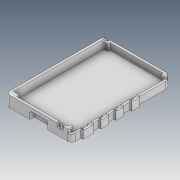
# Autodesk Inventor part: raspberry_pi_base
Saved by Autodesk Inventor 2020 (Build 240168000, 168)
## iProperties
Created: 2020-10-02
Part Number: raspberry_pi_base
Material: Generic
Document SubType Name: Modeling
Designer: DELL
Density: 1 g/cm^3
Appearance: Default
Mass: 14.8212 g
Surface Area: 156.939 cm^2
Volume: 14.8212 cm^3
Author: DELL
Autodesk Inventor part; units mm, degrees
ref_plane "YZ Plane" through (0, 0, 0) normal (1, 0, 0) x (0, 1, 0)
ref_plane "XZ Plane" through (0, 0, 0) normal (0, 1, 0) x (-1, 0, 0)
ref_plane "XY Plane" through (0, 0, 0) normal (0, 0, 1) x (1, 0, 0)
sketch "Sketch1" plane through (0, 0, 0) normal (0, 1, 0) x (-1, 0, 0)
  line L0 (-26.5, -44.85) -> (26.5, -44.85)
  line L1 (30, -41.35) -> (30, 41.35)
  line L2 (26.5, 44.85) -> (-26.5, 44.85)
  line L3 (-30, 41.35) -> (-30, -41.35)
  line L4 (-30, -44.85) -> (30, 44.85) construction
  line L5 (30, -44.85) -> (-30, 44.85) construction
  arc A0 (30, 41.35) -> (26.5, 44.85) centre (26.5, 41.35) ccw
  arc A1 (-26.5, 44.85) -> (-30, 41.35) centre (-26.5, 41.35) ccw
  arc A2 (26.5, -44.85) -> (30, -41.35) centre (26.5, -41.35) ccw
  arc A3 (-30, -41.35) -> (-26.5, -44.85) centre (-26.5, -41.35) ccw
  line L6 (-26.4, -46.85) -> (26.4, -46.85)
  line L7 (26.4, -46.85) -> (26.4, 0)
  line L8 (26.4, 0) -> (-26.4, 0)
  line L9 (-26.4, 0) -> (-26.4, -46.85)
  line L10 (-26.4, -46.85) -> (26.4, 0) construction
  line L11 (26.4, -46.85) -> (-26.4, 0) construction
  point P0 (0, 0)
  point P1 (0, -23.425)
  point P2 (0, 0)
  point P3 (0, 0)
  point P4 (0, -23.425)
  point P5 (0, 0)
  point P6 (-26.4, -44.85)
  point P7 (26.4, -44.85)
  dimension "d0" = 89.7
  dimension "d1" = 60
  dimension "d2" = 3.5
  dimension "d3" = 2
  dimension "d4" = 52.8
  constraints: 24 end point, 8 midpoint, 8 point on circle, 8 point on line, 8 tangent, 4 centre point, 4 parallel, 3 equal radius, 2 horizontal, 2 perpendicular, 1 coincident, 1 vertical alignment
  measures "d0" distance of L5.start L4.end
  measures "d1" distance of L4.start L5.start
  measures "d2" radius of A0
  measures "d3" distance between parallel lines of L0 L6
  measures "d4" distance of L6.start L6.end
extrude "Extrusion1" add sketch "Sketch1" along normal blind 2
sketch "Sketch2" plane through (30, 0, 41.35) normal (1, 0, 0) x (0, 0, -1)
  line L0 (0, 0) -> (82.7, 0) projected
  line L1 (14.7, 0) -> (5.1, 0)
  line L2 (5.1, 8.5) -> (5.1, 8)
  line L3 (5.1, 8) -> (14.7, 8)
  line L4 (14.7, 8) -> (14.7, 8.5)
  line L5 (28.4, 0) -> (21.4, 0)
  line L6 (21.4, 0) -> (21.4, 8)
  line L7 (21.4, 8) -> (28.4, 8)
  line L8 (28.4, 8) -> (28.4, 0)
  line L9 (42.1, 0) -> (35.1, 0)
  line L10 (35.1, 0) -> (35.1, 8)
  line L11 (35.1, 8) -> (42.1, 8)
  line L12 (42.1, 8) -> (42.1, 0)
  line L13 (56.4, 0) -> (49.7, 0)
  line L14 (49.7, 0) -> (49.7, 9)
  line L15 (49.7, 9) -> (56.4, 9)
  line L16 (56.4, 9) -> (56.4, 0)
  line L17 (-3.5, 0) -> (-3.5, 2) projected
  line L18 (5.1, 8) -> (14.7, 8)
  line L19 (14.7, 8) -> (14.7, 7)
  line L20 (13.2, 7) -> (6.6, 7)
  line L21 (5.1, 7) -> (5.1, 8)
  arc A0 (5.1, 8.5) -> (6.6, 7) centre (6.6, 8.5) ccw
  arc A1 (13.2, 7) -> (14.7, 8.5) centre (13.2, 8.5) ccw
  line L22 (5.1, 7) -> (5.1, 0)
  line L23 (14.7, 7) -> (14.7, 0)
  line L24 (21.4, 8) -> (28.4, 8)
  line L25 (28.4, 8) -> (28.4, 8.5)
  line L26 (26.9, 7) -> (22.9, 7)
  line L27 (21.4, 8.5) -> (21.4, 8)
  arc A2 (21.4, 8.5) -> (22.9, 7) centre (22.9, 8.5) ccw
  arc A3 (26.9, 7) -> (28.4, 8.5) centre (26.9, 8.5) ccw
  line L28 (35.1, 8) -> (42.1, 8)
  line L29 (42.1, 8) -> (42.1, 8.5)
  line L30 (40.6, 7) -> (36.6, 7)
  line L31 (35.1, 8.5) -> (35.1, 8)
  arc A4 (35.1, 8.5) -> (36.6, 7) centre (36.6, 8.5) ccw
  arc A5 (40.6, 7) -> (42.1, 8.5) centre (40.6, 8.5) ccw
  arc A6 (49.7, 9) -> (56.4, 9) centre (53.05, 11.1857) ccw
  point P0 (41.35, 0)
  point P1 (35.1858, 8)
  point P2 (35.1, 0)
  point P3 (42.0142, 8)
  point P4 (21.4858, 8)
  point P5 (28.3142, 8)
  point P6 (14.7, 8)
  point P7 (14.6142, 8)
  point P8 (5.1858, 8)
  point P9 (5.1, 0)
  dimension "d7" = 8
  dimension "d8" = 9.6
  dimension "d9" = 8.6
  dimension "d10" = 1
  dimension "d11" = 1.5
  dimension "d12" = 6.7
  dimension "d13" = 7
  dimension "d14" = 1.5
  dimension "d15" = 1
  dimension "d16" = 6.7
  dimension "d17" = 1.5
  dimension "d18" = 1
  dimension "d19" = 7.6
  dimension "d20" = 6.7
  dimension "d21" = 9
  dimension "d22" = 8
  constraints: 60 end point, 15 parallel, 14 point on circle, 12 point on line, 12 tangent, 7 centre point, 7 horizontal, 7 perpendicular, 6 collinear, 3 equal radius, 1 vertical
  measures "d7" distance between parallel lines of L0 L3
  measures "d8" distance of L2.end L3.end
  measures "d9" distance between parallel lines of L17 L2
  measures "d10" distance between parallel lines of L3 L20
  measures "d11" radius of A0
  measures "d12" distance between parallel lines of L6 L23
  measures "d13" distance of L6.end L7.end
  measures "d14" radius of A2
  measures "d15" distance between parallel lines of L24 L26
  measures "d16" distance between parallel lines of L8 L10
  measures "d17" radius of A4
  measures "d18" distance between parallel lines of L28 L30
  measures "d19" distance between parallel lines of L12 L14
  measures "d20" distance of L14.end L15.end
  measures "d21" distance of L15.end L13.start
  measures "d22" diameter of A6
extrude "Extrusion2" add sketch "Sketch2" along normal blind 2 contours L22 L21 L3 A0 L20 A1 L19 L23 L0 | L14 A6 L16 L0 | L10 L11 A4 L30 A5 L12 L0 | L6 L7 A2 L26 A3 L8 L0
sketch "Sketch3" plane through (0, 2, 0) normal (0, 1, 0) x (1, 0, 0)
  line L0 (30, 15.05) -> (30, 41.35) projected
  arc A0 (30, 41.35) -> (26.5, 44.85) centre (26.5, 41.35) ccw projected
  line L1 (30, 15.05) -> (30, 8.35) projected
  line L2 (30, 0.75) -> (30, 8.35) projected
  line L3 (30, 0.6642) -> (30, -0.75) projected
  line L4 (30, -0.75) -> (30, -4.75) projected
  line L5 (30, -4.75) -> (30, -6.1642) projected
  line L6 (30, -12.95) -> (30, -6.25) projected
  line L7 (30, -13.0358) -> (30, -14.45) projected
  line L8 (30, -14.45) -> (30, -18.45) projected
  line L9 (30, -18.45) -> (30, -19.8642) projected
  line L10 (30, -26.65) -> (30, -19.95) projected
  line L11 (30, -26.7358) -> (30, -28.15) projected
  line L12 (30, -28.15) -> (30, -34.75) projected
  line L13 (30, -34.75) -> (30, -36.1642) projected
  line L14 (30, -41.35) -> (30, -36.25) projected
  arc A1 (26.5, -44.85) -> (30, -41.35) centre (26.5, -41.35) ccw projected
  arc A2 (28, 41.35) -> (26.5, 42.85) centre (26.5, 41.35) ccw
  line L15 (28, 41.35) -> (28, 15.05)
  line L16 (28, 8.35) -> (28, 0.75)
  line L17 (28, -36.25) -> (28, -41.35)
  arc A3 (26.5, -42.85) -> (28, -41.35) centre (26.5, -41.35) ccw
  line L18 (0, -42.85) -> (29.6623, -42.85)
  line L19 (-26.5, -44.85) -> (26.5, -44.85) projected
  line L20 (30, 10.45) -> (28, 10.45)
  line L21 (28, 12.95) -> (30, 12.95)
  line L22 (30, 10.45) -> (28, 12.95) construction
  line L23 (28, 10.45) -> (30, 12.95) construction
  line L24 (30, -4) -> (28, -4)
  line L25 (28, -1.5) -> (30, -1.5)
  line L26 (30, -4) -> (28, -1.5) construction
  line L27 (28, -4) -> (30, -1.5) construction
  line L28 (30, -17.7) -> (28, -17.7)
  line L29 (28, -15.2) -> (30, -15.2)
  line L30 (30, -17.7) -> (28, -15.2) construction
  line L31 (28, -17.7) -> (30, -15.2) construction
  line L32 (30, -34.2) -> (28, -34.2)
  line L33 (28, -28.7) -> (30, -28.7)
  line L34 (30, -31.45) -> (30, -34.2)
  line L35 (30, -34.2) -> (28, -28.7) construction
  line L36 (28, -34.2) -> (30, -28.7) construction
  line L37 (32, 8.35) -> (32, 15.05) construction
  line L38 (32, 11.7) -> (28, 11.7) construction
  line L39 (32, -6.25) -> (32, 0.75) construction
  line L40 (32, -2.75) -> (28, -2.75) construction
  line L41 (32, -14.45) -> (32, -18.45) construction
  line L42 (32, -16.45) -> (28, -16.45) construction
  line L43 (32, -36.25) -> (32, -26.65) construction
  line L44 (32, -31.45) -> (28, -31.45) construction
  line L45 (28, 15.05) -> (28, 12.95)
  line L46 (28, 10.45) -> (28, 8.35)
  line L47 (28, 0.75) -> (28, -1.5)
  line L48 (28, -4) -> (28, -15.2)
  line L49 (28, -17.7) -> (28, -28.7)
  line L50 (28, -34.2) -> (28, -36.25)
  line L51 (30, 10.45) -> (30, -1.5)
  line L52 (30, -4) -> (30, -15.2)
  line L53 (30, -17.7) -> (30, -28.7)
  line L54 (30, -34.2) -> (30, -41.35)
  line L55 (26.5, 42.85) -> (29.6623, 42.85)
  point P0 (0, 0)
  point P1 (29, 11.7)
  point P2 (29, -2.75)
  point P3 (29, -16.45)
  point P4 (29, -31.45)
  point P5 (29, 11.7)
  point P6 (29, -2.75)
  point P7 (29, -16.45)
  point P8 (29, -31.45)
  dimension "d25" = 2
  dimension "d27" = 2
  dimension "d28" = 2.5
  dimension "d29" = 2.5
  dimension "d30" = 2.5
  dimension "d31" = 5.5
  constraints: 72 end point, 18 midpoint, 8 horizontal, 7 point on circle, 6 collinear, 6 point on line, 4 parallel, 4 perpendicular, 2 centre point, 1 vertical, 2 other
  measures "d25" distance between parallel lines of L0 L15
  measures "d27" distance between parallel lines of L19 L18
  measures "d28" distance between parallel lines of L20 L21
  measures "d29" distance between parallel lines of L24 L25
  measures "d30" distance between parallel lines of L28 L29
  measures "d31" distance of L33.end L32.start
extrude "Extrusion3" add sketch "Sketch3" along normal blind 4.3
sketch "Sketch4" plane through (0, 2, 0) normal (0, 1, 0) x (1, 0, 0)
  line L0 (-26.4, 46.85) -> (-26.4, 44.85) projected
  line L1 (-26.4, 44.85) -> (-26.4, 46.85)
  line L2 (26.4, 46.85) -> (-26.4, 46.85) projected
  line L3 (-26.4, 46.85) -> (26.4, 46.85)
  line L4 (26.4, 46.85) -> (26.4, 44.85)
  arc A0 (-26.5, 44.85) -> (-30, 41.35) centre (-26.5, 41.35) ccw projected
  arc A1 (-26.5, 44.85) -> (-30, 41.35) centre (-26.5, 41.35) ccw
  line L5 (-26.4, 44.85) -> (-26.5, 44.85) projected
  line L6 (-26.5, 44.85) -> (-26.4, 44.85)
  line L7 (26.5, 44.85) -> (26.4, 44.85) projected
  line L8 (26.4, 44.85) -> (26.5, 44.85)
  line L9 (-26.5, 42.85) -> (-24.4, 42.85)
  line L10 (-24.4, 42.85) -> (-24.4, 44.85)
  line L11 (-24.4, 44.85) -> (24.4, 44.85)
  arc A2 (-26.5, 42.85) -> (-28, 41.35) centre (-26.5, 41.35) ccw
  line L12 (-30, 41.35) -> (-30, -41.35) projected
  line L13 (-30, 41.35) -> (-28, 41.35)
  line L14 (26.5, 42.85) -> (24.4, 42.85)
  arc A3 (28, 41.35) -> (26.5, 42.85) centre (26.5, 41.35) ccw projected
  line L15 (24.4, 42.85) -> (24.4, 44.85)
  arc A4 (29.6623, 42.85) -> (26.5, 44.85) centre (26.5, 41.35) ccw projected
  arc A5 (29.6623, 42.85) -> (26.5, 44.85) centre (26.5, 41.35) ccw
  line L16 (26.5, 42.85) -> (29.6623, 42.85)
  point P0 (0, 0)
  dimension "d35" = 2
  dimension "d36" = 2
  constraints: 24 end point, 6 point on circle, 3 centre point, 3 coincident, 3 collinear, 3 horizontal, 3 perpendicular, 1 tangent, 1 other
  measures "d35" distance between parallel lines of L0 L10
  measures "d36" distance between parallel lines of L4 L15
extrude "Extrusion4" add sketch "Sketch4" along normal blind 6
sketch "Sketch5" plane through (0, 2, 0) normal (0, 1, 0) x (1, 0, 0)
  arc A0 (-26.5, 44.85) -> (-30, 41.35) centre (-26.5, 41.35) ccw projected
  line L0 (-30, 41.35) -> (-30, -41.35) projected
  arc A1 (-30, -41.35) -> (-26.5, -44.85) centre (-26.5, -41.35) ccw projected
  line L1 (-26.5, -44.85) -> (26.5, -44.85) projected
  arc A2 (26.5, -44.85) -> (29.6623, -42.85) centre (26.5, -41.35) ccw projected
  arc A3 (26.5, -42.85) -> (27.8553, -41.9929) centre (26.5, -41.35) ccw
  line L2 (26.5, -42.85) -> (-26.5, -42.85)
  arc A4 (-28, -41.35) -> (-26.5, -42.85) centre (-26.5, -41.35) ccw
  line L3 (-28, -41.35) -> (-28, 41.35)
  arc A5 (-26.5, 42.85) -> (-28, 41.35) centre (-26.5, 41.35) ccw
  line L4 (29.6623, -42.85) -> (26.5, -42.85) projected
  line L5 (26.5, -42.85) -> (29.6623, -42.85)
  line L6 (-28, 41.35) -> (-28, 44.5123)
  point P0 (0, 0)
  dimension "d39" = 2
  constraints: 8 end point, 7 point on circle, 3 centre point, 1 horizontal, 1 vertical, 4 other
  measures "d39" distance between parallel lines of L1 L2
extrude "Extrusion5" add sketch "Sketch5" along normal blind 8
sketch "Sketch6" plane through (0, 10, 0) normal (0, 1, 0) x (1, 0, 0)
  line L0 (-28, 41.35) -> (-28, -41.35) projected
  line L1 (-28, -40.35) -> (-22.5, -40.35)
  line L2 (-22.5, -40.35) -> (-22.5, -42.85)
  line L3 (-26.5, -42.85) -> (26.5, -42.85) projected
  line L4 (-28, -41.35) -> (-28, 44.5123) projected
  arc A0 (-28, -41.35) -> (-26.5, -42.85) centre (-26.5, -41.35) ccw projected
  line L5 (29.6623, -42.85) -> (-26.5, -42.85) projected
  line L6 (-30, 41.35) -> (-30, -41.35) projected
  line L7 (-26.5, -44.85) -> (26.5, -44.85) projected
  point P0 (0, 0)
  dimension "d53" = 2.3
  dimension "d42" = 7.5
  dimension "d43" = 4.5
  constraints: 4 end point, 2 point on line, 1 horizontal, 1 perpendicular
  measures "d42" distance between parallel lines of L6 L2
  measures "d43" distance between parallel lines of L7 L1
extrude "Extrusion6" add sketch "Sketch6" against normal blind 1.5
sketch "Sketch7" plane through (0, 10, 0) normal (0, 1, 0) x (1, 0, 0)
  line L0 (27, -44.85) -> (27, -40.65)
  line L1 (27, -40.65) -> (24.7, -40.65)
  line L2 (24.7, -40.65) -> (24.7, -42.85)
  line L3 (24.7, -42.85) -> (22.8, -42.85)
  line L4 (22.8, -42.85) -> (22.8, -44.85)
  line L5 (22.8, -44.85) -> (27, -44.85)
  line L6 (30, -41.35) -> (30, -36.25) projected
  line L7 (-26.5, -44.85) -> (26.5, -44.85) projected
  point P0 (0, 0)
  dimension "d46" = 2.3
  dimension "d47" = 4.2
  dimension "d48" = 4.2
  dimension "d49" = 2
  dimension "d50" = 3
  constraints: 12 end point, 5 perpendicular, 1 collinear, 1 vertical
  measures "d46" distance of L0.end L1.end
  measures "d47" distance of L0.start L0.end
  measures "d48" distance of L4.end L0.start
  measures "d49" distance of L3.end L4.end
  measures "d50" distance between parallel lines of L6 L0
extrude "Extrusion7" add sketch "Sketch7" against normal blind 1.5
sketch "Sketch8" plane through (0, 10, 0) normal (0, 1, 0) x (1, 0, 0)
  line L0 (27, -42.85) -> (29.6623, -42.85)
  line L1 (29.6623, -42.85) -> (29.6623, -44.85)
  line L2 (29.6623, -44.85) -> (27, -44.85)
  line L3 (27, -44.85) -> (27, -42.85)
  line L4 (-26.5, -44.85) -> (27, -44.85) projected
  line L5 (-26.5, -42.85) -> (26.5, -42.85) projected
  line L6 (16.8, -42.85) -> (19.1, -42.85)
  line L7 (19.1, -42.85) -> (19.1, -44.85)
  line L8 (19.1, -44.85) -> (16.8, -44.85)
  line L9 (16.8, -44.85) -> (16.8, -42.85)
  line L10 (-26.5, -44.85) -> (26.5, -44.85) projected
  line L11 (20.1, -42.85) -> (22.4, -42.85)
  line L12 (22.4, -42.85) -> (22.4, -44.85)
  line L13 (22.4, -44.85) -> (20.1, -44.85)
  line L14 (20.1, -44.85) -> (20.1, -42.85)
  line L15 (24.7, -40.65) -> (24.7, -42.85) projected
  point P0 (0, 0)
  dimension "d53" = 2.3
  dimension "d55" = 2.3
  dimension "d56" = 1
  dimension "d57" = 2.3
  constraints: 24 end point, 6 parallel, 5 point on line, 3 horizontal, 3 perpendicular, 1 collinear
  measures "d53" distance between parallel lines of L12 L15
  measures "d55" distance between parallel lines of L14 L12
  measures "d56" distance between parallel lines of L7 L14
  measures "d57" distance between parallel lines of L9 L7
extrude "Extrusion8" cut sketch "Sketch8" against normal up to surface (3.7 mm away) contours L4 L14 L5 L12 | L0 L1 L2 L3 | L4 L9 L5 L7
sketch "Sketch11" plane through (-26.5, 0, 44.85) normal (0, 0, 1) x (1, 0, 0)
  line L0 (52.9, 0) -> (0.1, 0) projected
  line L1 (33.2, 6.8) -> (19.8, 6.8)
  line L2 (18.3, 5.3) -> (18.3, 0)
  line L3 (18.3, 0) -> (34.7, 0)
  line L4 (34.7, 0) -> (34.7, 5.3)
  line L5 (34.7, 6.8) -> (18.3, 0) construction
  line L6 (18.3, 6.8) -> (34.7, 0) construction
  arc A0 (19.8, 6.8) -> (18.3, 5.3) centre (19.8, 5.3) ccw
  arc A1 (34.7, 5.3) -> (33.2, 6.8) centre (33.2, 5.3) ccw
  point P0 (26.5, 0)
  point P1 (26.5, 3.4)
  point P2 (26.5, 3.4)
  point P3 (26.5, 0)
  dimension "d71" = 6.8
  dimension "d72" = 16.4
  dimension "d73" = 1.5
  constraints: 12 end point, 5 point on line, 4 midpoint, 4 point on circle, 4 tangent, 2 centre point, 2 parallel, 1 equal radius, 1 horizontal, 1 perpendicular, 1 vertical alignment
  measures "d71" distance between parallel lines of L0 L1
  measures "d72" distance of L5.start L6.start
  measures "d73" radius of A0
extrude "Extrusion12" cut sketch "Sketch11" against normal blind 3.8
sketch "Sketch12" plane through (0, 2, 0) normal (0, 1, 0) x (1, 0, 0)
  line L0 (-8.2, -41.05) -> (8.2, -41.05) projected
  line L1 (-8.2, -42.85) -> (-8.2, -41.05) projected
  line L2 (8.2, -41.05) -> (8.2, -42.85) projected
  line L3 (9.2, -42.85) -> (9.2, -40.05)
  line L4 (9.2, -40.05) -> (-9.2, -40.05)
  line L5 (-9.2, -40.05) -> (-9.2, -42.85)
  line L6 (-8.2, -42.85) -> (-9.2, -42.85)
  line L7 (-9.2, -42.85) -> (-9.2, -38.05)
  line L8 (-9.2, -38.05) -> (-8.2, -38.05)
  line L9 (-8.2, -38.05) -> (-8.2, -42.85)
  line L10 (9.2, -42.85) -> (8.2, -42.85)
  line L11 (8.2, -42.85) -> (8.2, -38.05)
  line L12 (8.2, -38.05) -> (9.2, -38.05)
  line L13 (9.2, -38.05) -> (9.2, -42.85)
  line L14 (16.8, -42.85) -> (-22.5, -42.85) projected
  point P0 (0, 0)
  point P1 (8.2, -40.05)
  point P2 (-8.2, -40.05)
  dimension "d76" = 1
  dimension "d77" = 4.8
  constraints: 22 end point, 4 parallel, 3 collinear, 2 horizontal, 2 perpendicular, 2 other
  measures "d76" distance between parallel lines of L0 L4
  measures "d77" distance between parallel lines of L6 L8
extrude "Extrusion13" add sketch "Sketch12" along normal blind 2 contours L9 L4 L11 L0
extrude "Extrusion14" add sketch "Sketch12" along normal blind 3 contours L1 L6 L5 L4 L9 | L11 L4 L3 L10 L2 | L4 L7 L8 L9 | L11 L12 L13 L4
body "Solid1"
